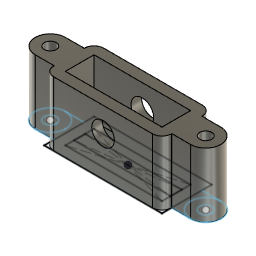
sd-card-thing (Autodesk Fusion 360 design; units mm, degrees)
Autodesk Fusion 360 part; units mm, degrees
sketch "Skizze1" plane through (0, 0, 0) normal (0, 0, 1) x (1, 0, 0)
  line L0 (12.8, 3.8) -> (-12.8, 3.8)
  line L1 (-12.8, 3.8) -> (-12.8, -3.8)
  line L2 (-12.8, -3.8) -> (12.8, -3.8)
  line L3 (12.8, -3.8) -> (12.8, 3.8)
  line L4 (12.8, 3.8) -> (-12.8, -3.8) construction
  line L5 (-12.8, 3.8) -> (12.8, -3.8) construction
  line L6 (-15.6, 6.6) -> (-15.6, -6.6)
  line L7 (-15.6, -6.6) -> (15.6, -6.6)
  line L8 (15.6, -6.6) -> (15.6, 6.6)
  line L9 (15.6, 6.6) -> (-15.6, 6.6)
  line L10 (12.8, 1.5) -> (-12.8, 1.5)
  line L11 (-12.8, 1.5) -> (-12.8, -1.5)
  line L12 (-12.8, -1.5) -> (12.8, -1.5)
  line L13 (12.8, -1.5) -> (12.8, 1.5)
  line L14 (12.8, 1.5) -> (-12.8, -1.5) construction
  line L15 (-12.8, 1.5) -> (12.8, -1.5) construction
  circle A0 centre (20.6, 0) radius 1.6
  circle A1 centre (-20.6, 0) radius 1.6
  circle A2 centre (20.6, 0) radius 4
  circle A3 centre (-20.6, 0) radius 4
  line L16 (-20.6, 4) -> (-15.6, 4)
  line L17 (-20.6, -4) -> (-15.6, -4)
  line L18 (20.6, 4) -> (15.6, 4)
  line L19 (20.6, -4) -> (15.6, -4)
  dimension "d1" = 25.6
  dimension "d2" = 7.6
  dimension "d3" = 2.8
  dimension "d4" = 3
  dimension "d5" = 3.2
  dimension "d6" = 5
  dimension "d7" = 3.2
  dimension "d8" = 5
  dimension "d9" = 8
  dimension "d10" = 8
  constraint horizontal L0
  constraint perpendicular L0 L1
  constraint parallel L0 L2
  constraint parallel L1 L3
  constraint coincident L4 origin
  constraint coincident L5 origin
  constraint horizontal L10
  constraint perpendicular L10 L11
  constraint parallel L10 L12
  constraint parallel L11 L13
  constraint coincident L3 L10.start
  constraint coincident L14 origin
  constraint coincident L15 origin
  constraint concentric A0 A2
  constraint concentric A1 A3
  constraint coincident A3 L16.start
  constraint coincident L6 L16.end
  constraint tangent A3 L16
  constraint perpendicular L6 L16
  constraint coincident A3 L17.start
  constraint coincident L6 L17.end
  constraint tangent A3 L17
  constraint perpendicular L6 L17
  constraint coincident A2 L18.start
  constraint coincident L8 L18.end
  constraint tangent A2 L18
  constraint perpendicular L8 L18
  constraint coincident A2 L19.start
  constraint coincident L8 L19.end
  constraint tangent A2 L19
  constraint perpendicular L8 L19
  measures "d1" distance of L1.end L2.end
  measures "d2" distance of L0.end L1.end
  measures "d4" distance of L10.end L11.end
  measures "d5" diameter of A0
  measures "d6" distance of L8 A0.centre
  measures "d7" diameter of A1
  measures "d8" distance of L6 A1.centre
  measures "d9" diameter of A2
  measures "d10" diameter of A3
extrude "Extrusion1" add sketch "Skizze1" along normal blind 4 contours L0 L1 L3 L10 | L1 L2 L3 L12 | L6 L7 L8 L9 | L6 A3 L16 L17 | A3 | L8 A2 L18 L19 | A2
sketch "Skizze2" plane through (0, 0, 4) normal (0, 0, 1) x (-1, 0, 0)
  circle A0 centre (-20.6, 0) radius 1.6
  line L0 (-12.8, -1.5) -> (-12.8, 1.5)
  line L1 (-12.8, 1.5) -> (12.8, 1.5)
  line L2 (12.8, 1.5) -> (12.8, -1.5)
  line L3 (12.8, -1.5) -> (-12.8, -1.5)
  circle A1 centre (20.6, 0) radius 1.6
  line L4 (-20.6, -4) -> (-15.6, -4)
  line L5 (-15.6, -4) -> (-15.6, -6.6)
  line L6 (-15.6, -6.6) -> (15.6, -6.6)
  line L7 (15.6, -6.6) -> (15.6, -4)
  line L8 (15.6, -4) -> (20.6, -4)
  arc A2 (20.6, -4) -> (20.6, 4) centre (20.6, 0) ccw
  line L9 (20.6, 4) -> (15.6, 4)
  line L10 (15.6, 4) -> (15.6, 6.6)
  line L11 (15.6, 6.6) -> (-15.6, 6.6)
  line L12 (-15.6, 6.6) -> (-15.6, 4)
  line L13 (-15.6, 4) -> (-20.6, 4)
  arc A3 (-20.6, 4) -> (-20.6, -4) centre (-20.6, 0) ccw
  line L14 (-12.8, -3.8) -> (12.8, -3.8)
  line L15 (12.8, -3.8) -> (12.8, 3.8)
  line L16 (12.8, 3.8) -> (-12.8, 3.8)
  line L17 (-12.8, 3.8) -> (-12.8, -3.8)
extrude "Extrusion2" add sketch "Skizze2" along normal blind 13
fillet "Abrundung1" radius 2 4 edges at (12.8, 2.65, 4) (12.8, -2.65, 4) (-12.8, -2.65, 4) (-12.8, 2.65, 4)
fillet "Abrundung2" radius 2.5 4 edges at (-15.6, -6.6, 8.5) (15.6, -6.6, 8.5) (15.6, 6.6, 8.5) (-15.6, 6.6, 8.5)
sketch "Skizze3" plane through (0, -6.6, 0) normal (0, -1, 0) x (1, 0, 0)
  line L0 (13.1, 0) -> (13.1, 17)
  line L1 (13.1, 17) -> (-13.1, 17)
  line L2 (-13.1, 17) -> (-13.1, 0)
  line L3 (-13.1, 0) -> (13.1, 0)
  circle A0 centre (0, 10.5) radius 3
  line L4 (5.8778, 17) -> (5.8778, 4) construction
  point P0 (5.8778, 10.5)
  dimension "d19" = 6
  constraint coincident L1 L4.start
  constraint perpendicular L1 L4
  constraint midpoint L4 P0
  constraint vertical A0.centre origin
  constraint horizontal A0.centre P0
  measures "d19" diameter of A0
extrude "Extrusion3" cut sketch "Skizze3" against normal up to surface (13.2 mm away) contours A0
